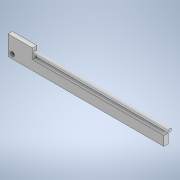
# Autodesk Inventor part: new bolt
Saved by Autodesk Inventor 2022 (Build 260153070, 153G)
## iProperties
Created: 2021-07-24
Part Number: new bolt
Material: Generic
Document SubType Name: Sheet Metal
Designer: DELL
Density: 1 g/cm^3
Sheet Metal Rule: Default
Appearance: Default
Author: DELL
Autodesk Inventor part; units mm, degrees
ref_plane "YZ Plane" through (0, 0, 0) normal (1, 0, 0) x (0, 1, 0)
ref_plane "XZ Plane" through (0, 0, 0) normal (0, 1, 0) x (-1, 0, 0)
ref_plane "XY Plane" through (0, 0, 0) normal (0, 0, 1) x (1, 0, 0)
sketch "Sketch1" plane through (0, 0, 0) normal (0, 0, 1) x (1, 0, 0)
  line L0 (0, 0) -> (457.2, 0)
  line L1 (457.2, 0) -> (457.2, 28.58)
  line L2 (457.2, 28.58) -> (72.12, 28.58)
  line L3 (0, 28.58) -> (0, 0)
  line L4 (0, 8.7151) -> (0, 28.58)
  line L5 (72.12, 28.58) -> (72.12, 57.5527)
  line L6 (72.12, 57.5527) -> (0, 57.5527)
  line L7 (0, 57.5527) -> (0, 28.58)
  dimension "d0" = 457.2
  dimension "d2" = 28.58
  dimension "d4" = 72.12
  constraints: 16 end point, 3 parallel, 1 horizontal, 1 perpendicular
  measures "d0" distance of L0.start L0.end
  measures "d2" distance from line of L2 L0.end
  measures "d4" distance between parallel lines of L5 L4
extrude "Extrusion1" add sketch "Sketch1" along normal blind 12.7
sketch "Sketch2" plane through (72.12, 28.58, 0) normal (1, 0, 0) x (0, 0, -1)
  circle A0 centre (-6.0784, 15.0544) radius 4.7759
  line L0 (0, 28.9727) -> (-12.7, 28.9727) projected
  line L1 (-12.7, 0) -> (-12.7, 28.9727) projected
  point P0 (0, -28.58)
  constraints: 1 centre point
extrude "Extrusion2" add sketch "Sketch2" along normal blind 396.0622
sketch "Sketch3" plane through (72.12, 28.58, 0) normal (0, 1, 0) x (1, 0, 0)
  point P0 (-72.12, 0)
sketch "Sketch4" plane through (0, 0, 12.7) normal (0, 0, 1) x (1, 0, 0)
  circle A0 centre (12.7, 12.7) radius 6.35
  line L0 (0, 0) -> (457.2, 0) projected
  line L1 (0, 57.5527) -> (0, 0) projected
  dimension "d12" = 12.7
  dimension "d13" = 12.7
  dimension "d14" = 12.7
  constraints: 1 centre point
  measures "d12" diameter of A0
  measures "d13" distance from line of L0 A0.centre
  measures "d14" distance from line of L1 A0.centre
hole "Hole1" at (12.7, 12.7, 12.7) direction (0, 0, -1) diameter 12.7 end through all
equation "\"d20\" = Thickness"
equation "\"BendRadius\" = Thickness"
equation "\"BendReliefWidth\" = Thickness"
equation "\"BendReliefDepth\" = 0.5 * Thickness"
equation "\"CornerReliefSize\" = 4 * Thickness"
equation "\"MinimumRemnant\" = 2 * Thickness"
equation "\"TransitionRadius\" = BendRadius"
equation "\"JacobiRadiusSize\" = BendRadius"
equation "\"GapSize\" = Thickness"
equation "\"Thickness\" = 3.048"
body "Solid1"
